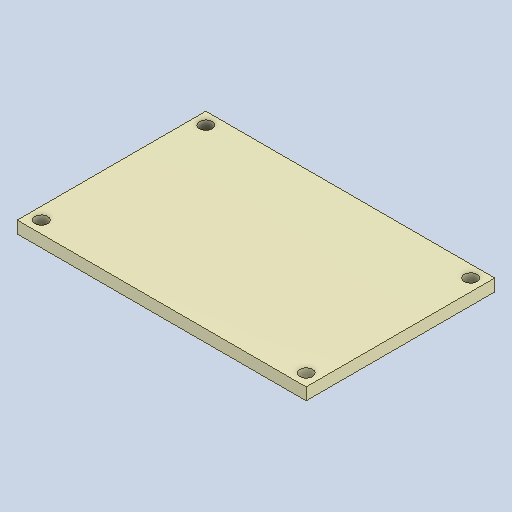
# Autodesk Inventor part: mainBoard
Saved by Autodesk Inventor 2022 (Build 260153000, 153)
## iProperties
Created: 2021-07-08
Part Number: mainBoard
Material: ポリプロピレン
Document SubType Name: Modeling
Designer: ken
Density: 0.899 g/cm^3
Appearance: 滑らか - 灰色
Author: ken
Autodesk Inventor part; units mm, degrees
ref_plane "YZ Plane" through (0, 0, 0) normal (1, 0, 0) x (0, 1, 0)
ref_plane "XZ Plane" through (0, 0, 0) normal (0, 1, 0) x (-1, 0, 0)
ref_plane "XY Plane" through (0, 0, 0) normal (0, 0, 1) x (1, 0, 0)
sketch "スケッチ1" plane through (0, 0, 0) normal (0, 1, 0) x (-1, 0, 0)
  line L0 (0, 0) -> (72, 0)
  line L1 (72, 0) -> (72, -47)
  line L2 (72, -47) -> (0, -47)
  line L3 (0, -47) -> (0, 0)
  dimension "d0" = 72
  dimension "d1" = 47
  constraints: 8 end point, 2 parallel, 1 horizontal, 1 perpendicular
  measures "d0" distance of L1.end L2.end
  measures "d1" distance of L0.end L1.end
extrude "押し出し1" add sketch "スケッチ1" along normal blind 3
sketch "スケッチ2" plane through (0, 3, 0) normal (0, 1, 0) x (1, 0, 0)
  line L0 (-72, 47) -> (-72, 0) projected
  line L1 (0, 47) -> (-72, 47) projected
  line L2 (-72, 0) -> (0, 0) projected
  line L3 (0, 0) -> (0, 47) projected
  point P0 (-69, 3)
  point P1 (-69, 44)
  point P2 (-3, 3)
  point P3 (-3, 44)
  dimension "d4" = 3
  dimension "d5" = 3
  dimension "d6" = 3
  dimension "d7" = 3
  dimension "d15" = 41
  dimension "d16" = 66
  constraints: 2 horizontal alignment, 2 vertical alignment
  measures "d4" distance from line of L0 point (-69, 44)
  measures "d5" distance from line of L1 point (-69, 44)
  measures "d6" distance from line of L2 point (-69, 3)
  measures "d7" distance from line of L3 point (-3, 3)
  measures "d15" distance of point (-69, 44) point (-69, 3)
  measures "d16" distance of point (-3, 44) point (-69, 44)
hole "穴1" at (-69, 3, -3) at (-69, 3, -44) at (-3, 3, -3) at (-3, 3, -44) direction (0, -1, 0) diameter 3.2 depth 3
